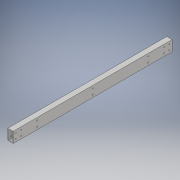
# Autodesk Inventor part: 1x2x30
Saved by Autodesk Inventor 2019 (Build 230136000, 136)
## iProperties
Created: 2018-11-11
Part Number: 1x2x30
Material: Generic
Document SubType Name: Modeling
Designer: maste
Density: 1 g/cm^3
Appearance: Default
Author: maste
Autodesk Inventor part; units mm, degrees
ref_plane "YZ Plane" through (0, 0, 0) normal (1, 0, 0) x (0, 1, 0)
ref_plane "XZ Plane" through (0, 0, 0) normal (0, 1, 0) x (-1, 0, 0)
ref_plane "XY Plane" through (0, 0, 0) normal (0, 0, 1) x (1, 0, 0)
sketch "Sketch1" plane through (0, 0, 0) normal (0, 0, 1) x (1, 0, 0)
  line L0 (0, 0) -> (25.4, 0)
  line L1 (25.4, 0) -> (25.4, 50.8)
  line L2 (25.4, 50.8) -> (0, 50.8)
  line L3 (0, 50.8) -> (0, 0)
  line L4 (22.225, 47.625) -> (22.225, 3.175)
  line L5 (22.225, 3.175) -> (3.175, 3.175)
  line L6 (3.175, 3.175) -> (3.175, 47.625)
  line L7 (3.175, 47.625) -> (22.225, 47.625)
  dimension "d0" = 25.4
  dimension "d1" = 50.8
  dimension "d2" = 3.175
  constraints: 16 end point, 4 parallel, 2 perpendicular, 1 horizontal, 3 other
  measures "d0" distance of L2.end L1.end
  measures "d1" distance of L1.end L0.end
  measures "d2" distance between parallel lines of L1 L4
extrude "Extrusion1" add sketch "Sketch1" along normal blind 762
sketch "Sketch2" plane through (25.4, 0, 0) normal (1, 0, 0) x (0, 0, -1)
  line L0 (0, 0) -> (-12.7, 0)
  line L1 (0, 0) -> (-762, 0) projected
  line L2 (-12.7, 0) -> (-12.7, 50.8)
  line L3 (0, 50.8) -> (-762, 50.8) projected
  line L4 (-12.7, 50.8) -> (-38.1, 50.8)
  line L5 (-38.1, 50.8) -> (-38.1, 0)
  line L6 (-12.7, 50.8) -> (-12.7, 38.1)
  line L7 (-12.7, 38.1) -> (-38.1, 38.1)
  line L8 (-38.1, 0) -> (-38.1, 12.7)
  line L9 (-38.1, 12.7) -> (-12.7, 12.7)
  circle A0 centre (-38.1, 38.1) radius 2.54
  circle A1 centre (-12.7, 38.1) radius 2.54
  circle A2 centre (-12.7, 12.7) radius 2.54
  circle A3 centre (-38.1, 12.7) radius 2.54
  line L10 (-381, 50.8) -> (-381, 0)
  line L11 (-762, 0) -> (-749.3, 0)
  line L12 (-762, 0) -> (0, 0)
  line L13 (-749.3, 0) -> (-749.3, 50.8)
  line L14 (-762, 50.8) -> (0, 50.8)
  line L15 (-749.3, 50.8) -> (-723.9, 50.8)
  line L16 (-723.9, 50.8) -> (-723.9, 0)
  line L17 (-749.3, 50.8) -> (-749.3, 38.1)
  line L18 (-749.3, 38.1) -> (-723.9, 38.1)
  line L19 (-723.9, 0) -> (-723.9, 12.7)
  line L20 (-723.9, 12.7) -> (-749.3, 12.7)
  circle A4 centre (-723.9, 38.1) radius 2.54
  circle A5 centre (-749.3, 38.1) radius 2.54
  circle A6 centre (-749.3, 12.7) radius 2.54
  circle A7 centre (-723.9, 12.7) radius 2.54
  dimension "d5" = 12.7
  dimension "d6" = 25.4
  dimension "d7" = 12.7
  dimension "d8" = 12.7
  dimension "d9" = 5.08
  dimension "d10" = 5.08
  dimension "d11" = 5.08
  dimension "d12" = 5.08
  constraints: 38 end point, 16 symmetric about line, 14 point on line, 8 centre point, 8 coincident, 5 perpendicular, 2 midpoint, 4 other
  measures "d5" distance of L0.start L0.end
  measures "d6" distance of L2.end L4.end
  measures "d7" distance of L2.end L6.end
  measures "d8" distance of L5.end L8.end
  measures "d9" diameter of A0
  measures "d10" diameter of A1
  measures "d11" diameter of A2
  measures "d12" diameter of A3
extrude "Extrusion2" cut sketch "Sketch2" against normal blind 762 contours A2 L9 L2 | L2 A2 | A3 L5 | L5 L9 A3 | L9 A2 L2 | L5 A3 L9 | A7 L20 L16 | L16 A7 | A0 L5 | L5 L7 A0 | A1 L7 L2 | L2 A1 | A6 L13 | L13 L20 A6 | L20 A7 L16 | A0 L7 L5 | A4 L16 | L16 L18 A4 | L7 A1 L2 | L13 A6 L20 | A5 L18 L13 | L13 A5 | L16 A4 L18 | L13 L18 A5
sketch "Sketch3" plane through (25.4, 0, 0) normal (1, 0, 0) x (0, 0, -1)
  line L0 (0, 0) -> (-114.3, 0)
  line L1 (0, 0) -> (-762, 0) projected
  line L2 (-114.3, 0) -> (-114.3, 50.8)
  line L3 (0, 50.8) -> (-762, 50.8) projected
  circle A0 centre (-114.3, 38.1) radius 2.54
  circle A1 centre (-114.3, 12.7) radius 2.54
  line L4 (0, 47.625) -> (-762, 47.625) projected
  line L5 (-381, 47.625) -> (-381, 0)
  circle A2 centre (-647.7, 38.1) radius 2.54
  circle A3 centre (-647.7, 12.7) radius 2.54
  circle A4 centre (-381, 38.1) radius 2.54
  circle A5 centre (-381, 12.7) radius 2.54
  dimension "d15" = 114.3
  dimension "d16" = 5.08
  constraints: 6 centre point, 6 end point, 6 point on line, 2 midpoint, 2 symmetric about line, 1 perpendicular, 2 other
  measures "d15" distance of L0.start L0.end
  measures "d16" diameter of A4
extrude "Extrusion3" cut sketch "Sketch3" against normal blind 25.4 contours A1 L2 | L2 A1 | A5 L5 | L5 A5 | A0 L2 | L2 A0 | A4 L5 | L5 A4 | A2 | A3
body "Solid1"
